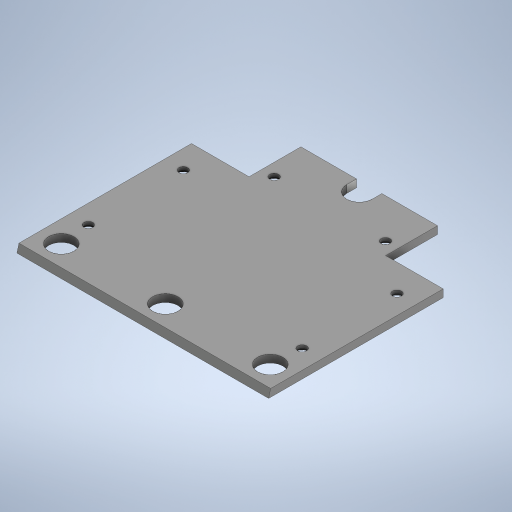
# Autodesk Inventor part: plech
Saved by Autodesk Inventor 2024 (Build 280153000, 153)
## iProperties
Created: 2023-11-08
Part Number: plech
Material: Všeobecné
Document SubType Name: Modeling
Designer: Simak
Density: 1 g/cm^3
Appearance: Výchozí
Author: Simak
Autodesk Inventor part; units mm, degrees
ref_plane "YZ Plane" through (0, 0, 0) normal (1, 0, 0) x (0, 1, 0)
ref_plane "XZ Plane" through (0, 0, 0) normal (0, 1, 0) x (-1, 0, 0)
ref_plane "XY Plane" through (0, 0, 0) normal (0, 0, 1) x (1, 0, 0)
sketch "Náčrt1" plane through (0, 0, 0) normal (0, 1, 0) x (-1, 0, 0)
  line L0 (49.75, -24.25) -> (49.75, 44.75)
  line L1 (49.75, 44.75) -> (-49.75, 44.75)
  line L2 (-49.75, 44.75) -> (-49.75, -24.25)
  line L3 (-49.75, -24.25) -> (-27, -24.25)
  line L4 (-27, -24.25) -> (-27, -44.75)
  line L5 (-27, -44.75) -> (27, -44.75)
  line L6 (27, -44.75) -> (27, -24.25)
  line L7 (27, -24.25) -> (49.75, -24.25)
  line L8 (49.75, -44.75) -> (0, 0) construction
  line L9 (0, 0) -> (-49.75, -44.75) construction
  line L10 (49.75, 44.75) -> (0, 0) construction
  line L11 (-49.75, 44.75) -> (0, 0) construction
  dimension "d0" = 99.5
  dimension "d1" = 89.5
  dimension "d2" = 20.5
  dimension "d3" = 54
  constraints: 24 end point, 6 perpendicular, 5 equal length, 2 horizontal alignment, 1 horizontal, 1 parallel, 1 vertical alignment
  measures "d0" distance of L0.end L1.end
  measures "d1" distance between parallel lines of L1 L5
  measures "d2" distance of L3.end L4.end
  measures "d3" distance of L4.end L5.end
extrude "Vysunutí1" add sketch "Náčrt1" along normal blind 3
sketch "Náčrt2" plane through (0, 3, 0) normal (0, 1, 0) x (1, 0, 0)
  circle A0 centre (0, -35.833) radius 5
  circle A1 centre (41.463, -35.833) radius 5
  circle A2 centre (-41.136, -35.833) radius 5
  circle A3 centre (0, 40.875) radius 5
  line L0 (49.75, -44.75) -> (49.75, 24.25) projected
  line L1 (-49.75, 24.25) -> (-49.75, -44.75) projected
  line L2 (-49.75, -44.75) -> (49.75, -44.75) projected
  line L3 (27, 44.75) -> (-27, 44.75) projected
  line L4 (-5, 40.875) -> (-5, 44.75)
  line L5 (5, 40.875) -> (5, 44.75)
  point P0 (0, 0)
  point P1 (3.1598, 44.75)
  point P2 (-3.1598, 44.75)
  dimension "d6" = 10
  dimension "d7" = 8.287
  dimension "d8" = 8.614
  dimension "d9" = 8.917
  dimension "d10" = 3.875
  constraints: 4 centre point, 4 end point, 3 equal radius, 2 horizontal alignment, 2 perpendicular, 2 point on circle, 2 point on line, 2 tangent, 2 vertical alignment
  measures "d6" diameter of A3
  measures "d7" distance from line of L0 A1.centre
  measures "d8" distance from line of L1 A2.centre
  measures "d9" distance from line of L2 A0.centre
  measures "d10" distance from line of A3.centre L3
extrude "Vysunutí2" cut sketch "Náčrt2" against normal through all
sketch "Náčrt3" plane through (49.75, 0, 44.75) normal (1, 0, 0) x (0, 0, -1)
  line L0 (0, 0) -> (69, 0) projected
  line L1 (0, 0) -> (0.8038, 3)
  line L2 (69, 3) -> (0, 3) projected
  line L3 (0, 0) -> (0, 3) projected
  point P0 (44.75, 0)
  dimension "d13" = 75
  constraints: 2 end point, 1 point on line
  measures "d13" angle of L0 L1
extrude "Vysunutí3" cut sketch "Náčrt3" against normal through all
sketch "Náčrt4" plane through (0, 0, 0) normal (0, -1, 0) x (1, 0, 0)
  line L0 (49.75, -24.25) -> (27, -24.25) projected
  line L1 (49.75, 44.75) -> (49.75, -24.25) projected
  line L2 (-49.75, -24.25) -> (-49.75, 44.75) projected
  line L3 (-27, -44.75) -> (-27, -24.25) projected
  line L4 (27, -24.25) -> (27, -44.75) projected
  point P0 (0, 0)
  point P1 (42.25, -13.5)
  point P2 (-42.25, -13.5)
  point P3 (42.25, 24)
  point P4 (-42.25, 24)
  point P5 (22, -29.1875)
  point P6 (-22, -29.1875)
  dimension "d16" = 10.75
  dimension "d17" = 7.5
  dimension "d18" = 7.5
  dimension "d19" = 37.5
  dimension "d27" = 5
  dimension "d28" = 5
  dimension "d29" = 4.9375
  constraints: 3 horizontal alignment, 2 vertical alignment
  measures "d16" distance from line of L0 point (42.25, -13.5)
  measures "d17" distance from line of L1 point (42.25, -13.5)
  measures "d18" distance from line of L2 point (-42.25, -13.5)
  measures "d19" distance of point (42.25, -13.5) point (42.25, 24)
  measures "d27" distance from line of L3 point (-22, -29.188)
  measures "d28" distance from line of L4 point (22, -29.188)
  measures "d29" distance from line of point (22, -29.188) L0
hole "Díra1" at (-42.25, 0, -13.5) at (-42.25, 0, 24) at (42.25, 0, 24) at (42.25, 0, -13.5) at (22, 0, -29.1875) at (-22, 0, -29.1875) direction (0, 1, 0) diameter 3.5 end through all countersink diameter 7 countersink angle 90
